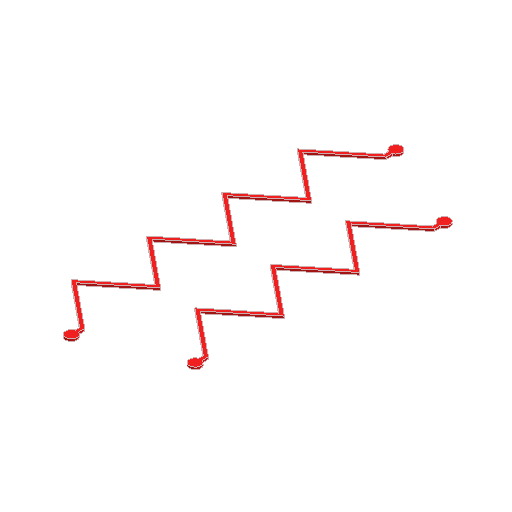
# Autodesk Inventor part: Serpentine
Saved by Autodesk Inventor 2025.4 (Build 294407000, 407)
## iProperties
Created: 2026-04-28
Part Number: Serpentine
Material: Generic
Document SubType Name: Modeling
Designer: gdira
Density: 1 g/cm^3
Appearance: Default
Author: gdira
Autodesk Inventor part; units mm, degrees
ref_plane "YZ Plane" through (0, 0, 0) normal (1, 0, 0) x (0, 1, 0)
ref_plane "XZ Plane" through (0, 0, 0) normal (0, 1, 0) x (-1, 0, 0)
ref_plane "XY Plane" through (0, 0, 0) normal (0, 0, 1) x (1, 0, 0)
sketch "Sketch1" plane through (0, 0, 0) normal (0, 1, 0) x (-1, 0, 0)
  line L0 (872.3588, -264.5367) -> (891.8047, -264.5367)
  line L1 (891.8047, -199.5367) -> (874.1834, -199.5367)
  line L2 (874.1834, -232.0367) -> (891.8047, -232.0367)
  line L3 (889.426, -248.2867) -> (871.8047, -248.2867)
  line L4 (889.426, -215.7867) -> (871.8047, -215.7867)
  line L5 (874.1834, -134.5367) -> (891.8047, -134.5367)
  line L6 (874.1834, -167.0367) -> (891.8047, -167.0367)
  line L7 (889.426, -150.7867) -> (871.8047, -150.7867)
  line L8 (889.426, -183.2867) -> (871.8047, -183.2867)
  line L9 (872.3588, -264.0865) -> (891.8047, -248.2867)
  line L10 (890.6154, -247.3204) -> (870.8588, -263.3726)
  line L11 (890.6154, -247.3204) -> (871.8047, -232.0367)
  line L12 (872.9941, -231.0704) -> (892.7506, -247.1226)
  line L13 (891.8047, -215.7867) -> (872.9941, -231.0704)
  line L14 (870.8588, -230.8726) -> (890.6154, -214.8204)
  line L15 (890.6154, -214.8204) -> (871.8047, -199.5367)
  line L16 (872.9941, -198.5704) -> (892.7506, -214.6226)
  line L17 (872.9941, -198.5704) -> (891.8047, -183.2867)
  line L18 (890.6154, -182.3204) -> (870.8588, -198.3726)
  line L19 (890.6154, -182.3204) -> (871.8047, -167.0367)
  line L20 (872.7506, -165.8726) -> (892.7506, -182.1226)
  line L21 (872.9941, -166.0704) -> (891.8047, -150.7867)
  line L22 (890.6154, -149.8204) -> (870.8588, -165.8726)
  line L23 (890.6154, -149.8204) -> (871.8047, -134.5367)
  line L24 (872.3588, -133.8548) -> (872.7506, -133.3726)
  line L25 (873.3047, -133.8228) -> (892.7506, -149.6226)
  line L26 (871.8047, -134.5367) -> (871.8047, -129.5367)
  line L27 (871.8047, -129.5367) -> (872.3588, -129.5367)
  line L28 (873.3047, -129.5367) -> (873.3047, -133.8228)
  line L29 (872.3588, -134.5367) -> (871.8047, -134.5367)
  line L30 (870.8588, -263.3726) -> (870.8588, -265.9877)
  line L31 (870.8588, -268.3726) -> (872.3588, -268.3726)
  line L32 (872.3588, -265.9877) -> (872.3588, -264.0865)
  line L33 (871.8047, -263.3726) -> (870.8588, -263.3726)
  arc A0 (870.8588, -265.9877) -> (872.3588, -265.9877) centre (871.6088, -268.3726) ccw
  arc A1 (873.3047, -131.9216) -> (871.8047, -131.9216) centre (872.5547, -129.5367) ccw
  line L34 (891.8047, -248.2867) -> (892.9941, -247.3204)
  line L35 (891.8047, -246.354) -> (892.9941, -247.3204)
  line L36 (871.8047, -232.0367) -> (870.6154, -231.0704)
  line L37 (870.6154, -231.0704) -> (870.8588, -230.8726)
  line L38 (891.2024, -216.2761) -> (892.9941, -214.8204)
  line L39 (892.6168, -214.5138) -> (892.9941, -214.8204)
  line L40 (872.3588, -199.987) -> (870.3719, -198.3726)
  line L41 (871.8047, -197.604) -> (870.6154, -198.5704)
  line L42 (891.2024, -183.7761) -> (893.3444, -182.0358)
  line L43 (891.711, -181.2778) -> (892.9941, -182.3204)
  line L44 (872.8965, -167.9238) -> (870.6154, -166.0704)
  line L45 (870.6154, -166.0704) -> (871.8047, -165.104)
  line L46 (890.6154, -151.7531) -> (892.9941, -149.8204)
  line L47 (892.9941, -149.8204) -> (891.8047, -148.854)
  line L48 (891.8047, -148.854) -> (891.8047, -134.5367)
  line L49 (891.8047, -181.354) -> (891.8047, -150.7867)
  line L50 (871.8047, -134.5367) -> (871.8047, -165.104)
  line L51 (871.8047, -167.0367) -> (871.8047, -197.604)
  line L52 (891.8047, -213.854) -> (891.8047, -183.2867)
  line L53 (871.8047, -199.5367) -> (871.8047, -230.104)
  line L54 (871.8047, -232.0367) -> (871.8047, -262.604)
  line L55 (891.8047, -264.5367) -> (891.8047, -248.2867)
  line L56 (891.8047, -246.354) -> (891.8047, -215.7867)
  line L57 (891.8047, -134.5367) -> (874.1834, -134.5367)
  line L58 (872.3588, -134.5367) -> (871.8047, -134.5367)
  line L59 (835.1699, -248.1316) -> (854.6158, -248.1316)
  line L60 (854.6158, -183.1316) -> (836.9945, -183.1316)
  line L61 (836.9945, -215.6316) -> (854.6158, -215.6316)
  line L62 (852.2371, -231.8816) -> (834.6158, -231.8816)
  line L63 (852.2371, -199.3816) -> (834.6158, -199.3816)
  line L64 (852.2371, -166.8816) -> (834.6158, -166.8816)
  line L65 (835.1699, -247.6814) -> (854.6158, -231.8816)
  line L66 (853.4264, -230.9152) -> (833.6699, -246.9674)
  line L67 (853.4264, -230.9152) -> (834.6158, -215.6316)
  line L68 (835.8052, -214.6652) -> (855.5617, -230.7174)
  line L69 (854.6158, -199.3816) -> (835.8052, -214.6652)
  line L70 (833.6699, -214.4674) -> (853.4264, -198.4152)
  line L71 (853.4264, -198.4152) -> (834.6158, -183.1316)
  line L72 (835.8052, -182.1652) -> (855.5617, -198.2174)
  line L73 (835.8052, -182.1652) -> (854.6158, -166.8816)
  line L74 (853.4264, -165.9152) -> (833.6699, -181.9674)
  line L75 (853.4264, -165.9152) -> (834.6158, -150.6316)
  line L76 (835.5617, -149.4674) -> (855.5617, -165.7174)
  line L77 (833.6699, -246.9674) -> (833.6699, -249.5826)
  line L78 (833.6699, -251.9674) -> (835.1699, -251.9674)
  line L79 (835.1699, -249.5826) -> (835.1699, -247.6814)
  line L80 (834.6158, -246.9674) -> (833.6699, -246.9674)
  arc A2 (833.6699, -249.5826) -> (835.1699, -249.5826) centre (834.4199, -251.9674) ccw
  line L81 (854.6158, -231.8816) -> (855.8052, -230.9152)
  line L82 (854.6158, -229.9489) -> (855.8052, -230.9152)
  line L83 (834.6158, -215.6316) -> (833.4264, -214.6652)
  line L84 (833.4264, -214.6652) -> (833.6699, -214.4674)
  line L85 (854.0135, -199.8709) -> (855.8052, -198.4152)
  line L86 (855.4278, -198.1086) -> (855.8052, -198.4152)
  line L87 (835.1699, -183.5818) -> (833.183, -181.9674)
  line L88 (834.6158, -181.1989) -> (833.4264, -182.1652)
  line L89 (854.0135, -167.3709) -> (856.1555, -165.6306)
  line L90 (854.522, -164.8727) -> (855.8052, -165.9152)
  line L91 (854.6158, -164.9489) -> (854.6158, -134.3816)
  line L92 (834.6158, -150.6316) -> (834.6158, -181.1989)
  line L93 (854.6158, -197.4489) -> (854.6158, -166.8816)
  line L94 (834.6158, -183.1316) -> (834.6158, -213.6989)
  line L95 (834.6158, -215.6316) -> (834.6158, -246.1989)
  line L96 (854.6158, -248.1316) -> (854.6158, -231.8816)
  line L97 (854.6158, -229.9489) -> (854.6158, -199.3816)
  line L98 (835.1699, -150.6316) -> (836.1158, -150.6316)
  line L99 (836.1158, -149.9176) -> (836.1158, -148.0164)
  line L100 (836.1158, -145.6316) -> (834.6158, -145.6316)
  line L101 (834.6158, -148.0164) -> (834.6158, -150.6316)
  arc A3 (836.1158, -148.0164) -> (834.6158, -148.0164) centre (835.3658, -145.6316) ccw
  point P0 (891.7246, -181.2889)
  point P1 (816.0772, -65.3291)
  dimension "d38" = 20
  dimension "d42" = 1.5
  dimension "d45" = 1.5
  dimension "d47" = 1.5
  dimension "d48" = 5
  dimension "d49" = 1.5
  dimension "d50" = 5
  dimension "d51" = 1.5
  dimension "d52" = 5
  dimension "d53" = 5
  dimension "d55" = 1.5
  dimension "d56" = 1.5
  dimension "d60" = 5
  dimension "d61" = 1.5
  dimension "d62" = 5
  dimension "d64" = 1.5
  dimension "d65" = 5
  dimension "d66" = 5
  dimension "d67" = 106.3358
  constraints: 204 end point, 74 point on line, 56 parallel, 16 perpendicular, 10 symmetric about line, 8 point on circle, 4 centre point, 3 horizontal, 3 midpoint
  measures "d38" distance of L5.end L23.end
  measures "d42" distance of L11.end L14.start
  measures "d45" distance of L19.end L20.start
  measures "d47" distance of L23.end L24.end
  measures "d48" distance of L23.end L26.end
  measures "d49" distance of L26.end L28.start
  measures "d50" distance of L10.end L31.start
  measures "d51" distance of L31.end L31.start
  measures "d52" diameter of A0
  measures "d53" diameter of A1
  measures "d55" distance of L95.start L70.start
  measures "d56" distance of L75.end L76.start
  measures "d60" distance of L66.end L78.start
  measures "d61" distance of L78.end L78.start
  measures "d62" diameter of A2
  measures "d64" distance of L75.end L98.end
  measures "d65" distance of L100.start L98.end
  measures "d66" diameter of A3
  measures "d67" vertical distance of L100.end L78.end
extrude "Extrusion1" add sketch "Sketch1" along normal blind 1 contours L32 A0 L30 L10 L11 L36 L37 L14 L15 L40 L41 L18 L19 L44 L45 L22 L23 L26 A1 L28 L25 L47 L46 L21 L20 L43 L42 L17 L16 L39 L38 L13 L12 L35 L34 L9 | L79 A2 L77 L66 L67 L83 L84 L70 L71 L87 L88 L74 L75 L101 A3 L99 L76 L90 L89 L73 L72 L86 L85 L69 L68 L82 L81 L65
body "Solid1"
